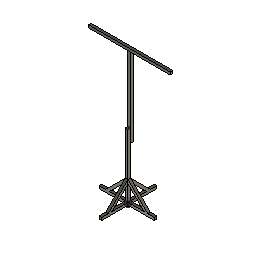
sensor_frame (Autodesk Fusion 360 design; units mm, degrees)
Autodesk Fusion 360 part; units mm, degrees
sketch "Sketch1" plane through (0, 0, 0) normal (0, 0, 1) x (1, 0, 0)
  line L0 (0, 0) -> (20, 0)
  line L1 (20, 0) -> (20, 20)
  line L2 (20, 20) -> (0, 20)
  line L3 (0, 20) -> (0, 0)
  line L4 (20, 20) -> (0, 0) construction
  line L5 (0, 20) -> (20, 0) construction
  point P0 (10, 10)
  dimension "d1" = 20
  dimension "d2" = 20
  constraint horizontal L0
  constraint vertical L1
  constraint horizontal L2
  constraint vertical L3
  constraint coincident L0.start L3.end
  constraint coincident L5 P0
  constraint coincident L4 P0
  measures "d1" distance of L0.start L0.end
  measures "d2" distance of L0.start L2.end
extrude "Extrude1" add sketch "Sketch1" along normal blind 500 makes body 1
sketch "Sketch2" plane through (20, 0, 0) normal (1, 0, 0) x (0, 0, -1)
  line L0 (0, 0) -> (0, 20)
  line L1 (0, 20) -> (-500, 20)
  line L2 (-500, 20) -> (-500, 0)
  line L3 (-500, 0) -> (0, 0)
  line L4 (0, 20) -> (-20, 20)
  line L5 (-20, 20) -> (-20, 220)
  line L6 (-20, 220) -> (0, 220)
  line L7 (0, 220) -> (0, 20)
  line L8 (-170, 20) -> (-20, 170)
  line L9 (-20, 141.7157) -> (-141.7157, 20)
  dimension "d5" = 20
  dimension "d6" = 200
  dimension "d7" = 20
  dimension "d8" = 45
  dimension "d9" = 50
  constraint horizontal L4
  constraint vertical L5
  constraint horizontal L6
  constraint vertical L7
  constraint coincident L0.end L1.start
  constraint coincident L1 L8.start
  constraint coincident L5 L8.end
  constraint coincident L5 L9.start
  constraint coincident L1 L9.end
  constraint parallel L8 L9
  measures "d5" distance of L0.end L4.end
  measures "d6" distance of L0.end L6.end
  measures "d7" distance of L8 L9
  measures "d8" angle of L5 L9
  measures "d9" distance of L5.end L8.end
extrude "Extrude2" add sketch "Sketch2" against normal blind 20 separate body contours L1 L4 L5 L6 L7 | L1 L5 L8 L9 makes body 2
pattern_circular "C-Pattern1" count 4 over 360 about axis through (10, 10, -20) along (0, 0, 1) of bodies 2 makes body 3 at (-107.2386, 20, 6.6667) makes body 4 at (0, -107.2386, 6.6667) makes body 5 at (127.2386, 0, 6.6667)
sketch "Sketch3" plane through (0, 0, 500) normal (0, 0, 1) x (1, 0, 0)
  line L0 (0, 20) -> (0, 0)
  line L1 (0, 0) -> (20, 0)
  line L2 (20, 0) -> (20, 20)
  line L3 (20, 20) -> (0, 20)
  line L4 (0, 0) -> (-20, 0)
  line L5 (-20, 0) -> (-20, 20)
  line L6 (-20, 20) -> (0, 20)
  line L7 (0, 20) -> (0, 0)
  constraint horizontal L4
  constraint vertical L5
  constraint horizontal L6
  constraint vertical L7
  constraint coincident L0.end L1.start
  constraint equal L5 L6
  constraint collinear L3 L6
extrude "Extrude3" add sketch "Sketch3" along normal blind 500 and the other way blind 100 separate body contours L0 L4 L5 L6 L7 makes body 6
sketch "Sketch4" plane through (0, 0, 0) normal (0, -1, 0) x (1, 0, 0)
  line L0 (0, 400) -> (0, 1000)
  line L1 (0, 1000) -> (-20, 1000)
  line L2 (-20, 1000) -> (-20, 400)
  line L3 (-20, 400) -> (0, 400)
  line L4 (-20, 1000) -> (0, 1000)
  line L5 (0, 1000) -> (0, 1020)
  line L6 (0, 1020) -> (-20, 1020)
  line L7 (-20, 1020) -> (-20, 1000)
  constraint horizontal L4
  constraint vertical L5
  constraint horizontal L6
  constraint vertical L7
  constraint coincident L1.end L2.start
  constraint equal L5 L6
  constraint collinear L0 L5
extrude "Extrude4" add sketch "Sketch4" along normal blind 300 and the other way blind 320 separate body contours L1 L4 L5 L6 L7 makes body 7
